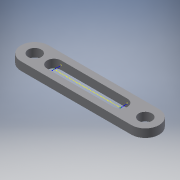
# Autodesk Inventor part: slider_link_p1
Saved by Autodesk Inventor 2017 (Build 210142000, 142)
## iProperties
Created: 2018-02-05
Part Number: slider_link_p1
Material: Generic
Document SubType Name: Modeling
Designer: Nic
Density: 1 g/cm^3
Appearance: Default
Author: Nic
Autodesk Inventor part; units mm, degrees
ref_plane "YZ Plane" through (0, 0, 0) normal (1, 0, 0) x (0, 1, 0)
ref_plane "XZ Plane" through (0, 0, 0) normal (0, 1, 0) x (-1, 0, 0)
ref_plane "XY Plane" through (0, 0, 0) normal (0, 0, 1) x (1, 0, 0)
sketch "Sketch1" plane through (0, 0, 0) normal (0, 0, 1) x (1, 0, 0)
  circle A0 centre (0, 0) radius 2.375
  circle A1 centre (40, 0) radius 2.375
  line L0 (0, 5) -> (40, 5)
  arc A2 (40, -5) -> (40, 5) centre (40, 0) ccw
  line L1 (40, -5) -> (0, -5)
  arc A3 (0, 5) -> (0, -5) centre (0, 0) ccw
  arc A4 (7, 2.55) -> (7, -2.55) centre (7, 0) ccw
  arc A5 (31, -2.55) -> (31, 2.55) centre (31, 0) ccw
  line L2 (7, 2.55) -> (31, 2.55)
  line L3 (31, -2.55) -> (7, -2.55)
  dimension "d1" = 4.75
  dimension "d2" = 40
  dimension "d3" = 5
  dimension "d7" = 5.1
  dimension "d8" = 7
  dimension "d9" = 9
  constraints: 8 end point, 8 point on circle, 8 tangent, 6 centre point, 3 equal radius, 3 horizontal alignment, 2 concentric, 1 coincident
  measures "d1" diameter of A1
  measures "d2" distance of point (0, 0) A1.centre
  measures "d3" radius of A2
  measures "d7" diameter of A4
  measures "d8" distance of point (0, 0) A4.centre
  measures "d9" distance of A1.centre A5.centre
extrude "Extrusion1" add sketch "Sketch1" along normal blind 3
sketch3d "3D Sketch1"
body "Solid1"
